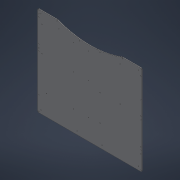
# Autodesk Inventor part: riglt_plate_01
Saved by Autodesk Inventor 2022 (Build 260153000, 153)
## iProperties
Created: 2025-01-09
Part Number: riglt_plate_01
Material: 一般
Document SubType Name: Modeling
Designer: nyxeon
Density: 1 g/cm^3
Appearance: 既定
Author: nyxeon
Autodesk Inventor part; units mm, degrees
ref_plane "YZ Plane" through (0, 0, 0) normal (1, 0, 0) x (0, 1, 0)
ref_plane "XZ Plane" through (0, 0, 0) normal (0, 1, 0) x (-1, 0, 0)
ref_plane "XY Plane" through (0, 0, 0) normal (0, 0, 1) x (1, 0, 0)
sketch "スケッチ1" plane through (0, 0, 0) normal (0, 0, 1) x (1, 0, 0)
  circle A0 centre (233.68, 2.54) radius 2.25 construction
  circle A1 centre (161.29, 2.54) radius 2.25 construction
  circle A2 centre (29.21, 2.54) radius 2.25 construction
  circle A3 centre (233.68, 160.02) radius 2.25 construction
  circle A4 centre (161.29, 160.02) radius 2.25 construction
  circle A5 centre (6.35, 160.02) radius 2.25 construction
  circle A6 centre (6.35, 284.48) radius 2.25 construction
  circle A7 centre (161.29, 284.48) radius 2.25 construction
  circle A8 centre (233.68, 284.48) radius 2.25 construction
  circle A9 centre (29.21, 2.54) radius 1.6
  circle A10 centre (161.29, 2.54) radius 1.6
  circle A11 centre (233.68, 2.54) radius 1.6
  circle A12 centre (233.68, 160.02) radius 1.6
  circle A13 centre (161.29, 160.02) radius 1.6
  circle A14 centre (6.35, 160.02) radius 1.6
  circle A15 centre (6.35, 284.48) radius 1.6
  circle A16 centre (161.29, 284.48) radius 1.6
  circle A17 centre (233.68, 284.48) radius 1.6
  line L0 (495.19, -98.01) -> (-14.81, -98.01)
  line L1 (-14.81, -98.01) -> (-14.81, 311.99)
  line L2 (-14.81, 311.99) -> (495.19, 311.99)
  line L3 (495.19, 311.99) -> (495.19, -98.01)
  line L4 (490.19, 306.99) -> (-9.81, 306.99) construction
  line L5 (-9.81, 306.99) -> (-9.81, -93.01) construction
  line L6 (-9.81, -93.01) -> (490.19, -93.01) construction
  line L7 (490.19, -93.01) -> (490.19, 306.99) construction
  circle A18 centre (-9.81, 306.99) radius 2.1
  circle A19 centre (490.19, 306.99) radius 2.1
  circle A20 centre (490.19, -93.01) radius 2.1
  circle A21 centre (-9.81, -93.01) radius 2.1
  circle A22 centre (-9.81, 6.99) radius 2.1
  circle A23 centre (-9.81, 106.99) radius 2.1
  circle A24 centre (-9.81, 206.99) radius 2.1
  circle A25 centre (90.19, 306.99) radius 2.1
  circle A26 centre (190.19, 306.99) radius 2.1
  circle A27 centre (290.19, 306.99) radius 2.1
  circle A28 centre (390.19, 306.99) radius 2.1
  line L8 (490.19, 106.99) -> (-9.81, 106.99) construction
  line L9 (240.19, -93.01) -> (240.19, 306.99) construction
  circle A29 centre (90.19, -93.01) radius 2.1
  circle A30 centre (190.19, -93.01) radius 2.1
  circle A31 centre (290.19, -93.01) radius 2.1
  circle A32 centre (390.19, -93.01) radius 2.1
  circle A33 centre (490.19, 6.99) radius 2.1
  circle A34 centre (490.19, 106.99) radius 2.1
  circle A35 centre (490.19, 206.99) radius 2.1
  point P0 (0, 0)
  point P1 (-3.81, 297.18)
  point P2 (0, 300.99)
  point P3 (3.7629, -59.9187)
  point P4 (-9.81, 106.99)
  dimension "d0" = 3.2
  dimension "d1" = 510
  dimension "d2" = 410
  dimension "d3" = 11
  dimension "d4" = 11
  dimension "d5" = 5
  dimension "d6" = 4.2
  dimension "d7" = 4.2
  dimension "d8" = 4.2
  dimension "d9" = 4.2
  dimension "d10" = 100
  dimension "d11" = 100
  dimension "d13" = 100
  dimension "d14" = 100
  dimension "d15" = 100
  dimension "d16" = 100
  dimension "d17" = 100
  dimension "d18" = 100
  dimension "d19" = 100
  dimension "d23" = 4.2
  dimension "d24" = 4.2
  dimension "d25" = 4.2
  dimension "d26" = 100
  dimension "d27" = 100
  dimension "d55" = 100
  constraints: 27 centre point, 20 end point, 19 equal radius, 13 coincident, 6 point on line, 5 horizontal alignment, 5 midpoint, 4 parallel, 4 vertical alignment, 2 perpendicular, 1 horizontal, 6 other
  measures "d0" diameter of A9
  measures "d1" distance of L1.end L2.end
  measures "d2" distance of L0.end L1.end
  measures "d3" distance from line of point (-3.81, 297.18) L1
  measures "d4" distance from line of L2 point (0, 300.99)
  measures "d5" distance between parallel lines of L2 L4
  measures "d6" diameter of A21
  measures "d7" diameter of A22
  measures "d8" diameter of A23
  measures "d9" diameter of A24
  measures "d10" distance of A22.centre L5.end
  measures "d11" distance of L8.end A22.centre
  measures "d13" distance of A18.centre A25.centre
  measures "d14" distance of A25.centre A26.centre
  measures "d15" distance of A26.centre A27.centre
  measures "d16" distance of A27.centre A28.centre
  measures "d17" distance of A29.centre A30.centre
  measures "d18" distance of A30.centre A31.centre
  measures "d19" distance of A31.centre A32.centre
  measures "d23" diameter of A33
  measures "d24" diameter of A34
  measures "d25" diameter of A35
  measures "d26" distance of A34.centre A33.centre
  measures "d27" distance of A35.centre A34.centre
  measures "d55" distance of A24.centre L8.end
extrude "押し出し1" add sketch "スケッチ1" along normal blind 3
fillet "フィレット1" radius 5 4 edges at (495.19, -98.01, 1.5) (-14.81, -98.01, 1.5) (-14.81, 311.99, 1.5) (495.19, 311.99, 1.5)
sketch "スケッチ2" plane through (0, 0, 3) normal (0, 0, 1) x (1, 0, 0)
  line L0 (-6.934, 160.0686) -> (-6.134, 160.0686) construction
  line L1 (-6.134, 160.0686) -> (-6.134, 170.6186) construction
  line L2 (-6.134, 170.6186) -> (-6.934, 170.6186) construction
  line L3 (-6.934, 170.6186) -> (-6.934, 160.0686) construction
  line L4 (-6.934, 159.9686) -> (-6.134, 159.9686) construction
  line L5 (-6.134, 170.7186) -> (-6.934, 170.7186)
  arc A0 (-7.334, 161.353) -> (-6.934, 159.9686) centre (-6.934, 160.7186) ccw
  line L6 (-5.734, 159.9686) -> (-5.734, 170.7186) construction
  arc A1 (-6.934, 170.7186) -> (-7.334, 169.3342) centre (-6.934, 169.9686) ccw
  line L7 (-7.334, 161.353) -> (-7.334, 169.3342)
  arc A2 (-6.134, 159.9686) -> (-6.134, 161.4686) centre (-6.134, 160.7186) ccw construction
  arc A3 (-6.134, 169.2186) -> (-6.134, 170.7186) centre (-6.134, 169.9686) ccw construction
  arc A4 (-6.134, 159.9686) -> (-5.734, 161.353) centre (-6.134, 160.7186) ccw
  arc A5 (-5.734, 169.3342) -> (-6.134, 170.7186) centre (-6.134, 169.9686) ccw
  line L8 (-5.734, 161.353) -> (-5.734, 169.3342)
  line L9 (-6.934, 159.9686) -> (-6.134, 159.9686)
  line L10 (-7.334, 181.753) -> (-7.334, 189.7342)
  arc A6 (-7.334, 181.753) -> (-6.934, 180.3686) centre (-6.934, 181.1186) ccw
  arc A7 (-6.134, 180.3686) -> (-5.734, 181.753) centre (-6.134, 181.1186) ccw
  line L11 (-5.734, 181.753) -> (-5.734, 189.7342)
  line L12 (-6.934, 180.3686) -> (-6.134, 180.3686)
  arc A8 (-6.934, 191.1186) -> (-7.334, 189.7342) centre (-6.934, 190.3686) ccw
  line L13 (-6.134, 191.1186) -> (-6.934, 191.1186)
  arc A9 (-5.734, 189.7342) -> (-6.134, 191.1186) centre (-6.134, 190.3686) ccw
  line L14 (-7.334, 202.153) -> (-7.334, 210.1342)
  arc A10 (-7.334, 202.153) -> (-6.934, 200.7686) centre (-6.934, 201.5186) ccw
  arc A11 (-6.134, 200.7686) -> (-5.734, 202.153) centre (-6.134, 201.5186) ccw
  line L15 (-5.734, 202.153) -> (-5.734, 210.1342)
  line L16 (-6.934, 200.7686) -> (-6.134, 200.7686)
  arc A12 (-6.934, 211.5186) -> (-7.334, 210.1342) centre (-6.934, 210.7686) ccw
  line L17 (-6.134, 211.5186) -> (-6.934, 211.5186)
  arc A13 (-5.734, 210.1342) -> (-6.134, 211.5186) centre (-6.134, 210.7686) ccw
  line L18 (-7.334, 222.553) -> (-7.334, 230.5342)
  arc A14 (-7.334, 222.553) -> (-6.934, 221.1686) centre (-6.934, 221.9186) ccw
  arc A15 (-6.134, 221.1686) -> (-5.734, 222.553) centre (-6.134, 221.9186) ccw
  line L19 (-5.734, 222.553) -> (-5.734, 230.5342)
  line L20 (-6.934, 221.1686) -> (-6.134, 221.1686)
  arc A16 (-6.934, 231.9186) -> (-7.334, 230.5342) centre (-6.934, 231.1686) ccw
  line L21 (-6.134, 231.9186) -> (-6.934, 231.9186)
  arc A17 (-5.734, 230.5342) -> (-6.134, 231.9186) centre (-6.134, 231.1686) ccw
  line L22 (-7.334, 242.953) -> (-7.334, 250.9342)
  arc A18 (-7.334, 242.953) -> (-6.934, 241.5686) centre (-6.934, 242.3186) ccw
  arc A19 (-6.134, 241.5686) -> (-5.734, 242.953) centre (-6.134, 242.3186) ccw
  line L23 (-5.734, 242.953) -> (-5.734, 250.9342)
  line L24 (-6.934, 241.5686) -> (-6.134, 241.5686)
  arc A20 (-6.934, 252.3186) -> (-7.334, 250.9342) centre (-6.934, 251.5686) ccw
  line L25 (-6.134, 252.3186) -> (-6.934, 252.3186)
  arc A21 (-5.734, 250.9342) -> (-6.134, 252.3186) centre (-6.134, 251.5686) ccw
  line L26 (-7.334, 263.353) -> (-7.334, 271.3342)
  arc A22 (-7.334, 263.353) -> (-6.934, 261.9686) centre (-6.934, 262.7186) ccw
  arc A23 (-6.134, 261.9686) -> (-5.734, 263.353) centre (-6.134, 262.7186) ccw
  line L27 (-5.734, 263.353) -> (-5.734, 271.3342)
  line L28 (-6.934, 261.9686) -> (-6.134, 261.9686)
  arc A24 (-6.934, 272.7186) -> (-7.334, 271.3342) centre (-6.934, 271.9686) ccw
  line L29 (-6.134, 272.7186) -> (-6.934, 272.7186)
  arc A25 (-5.734, 271.3342) -> (-6.134, 272.7186) centre (-6.134, 271.9686) ccw
  line L30 (-7.334, 283.753) -> (-7.334, 291.7342)
  arc A26 (-7.334, 283.753) -> (-6.934, 282.3686) centre (-6.934, 283.1186) ccw
  arc A27 (-6.134, 282.3686) -> (-5.734, 283.753) centre (-6.134, 283.1186) ccw
  line L31 (-5.734, 283.753) -> (-5.734, 291.7342)
  line L32 (-6.934, 282.3686) -> (-6.134, 282.3686)
  arc A28 (-6.934, 293.1186) -> (-7.334, 291.7342) centre (-6.934, 292.3686) ccw
  line L33 (-6.134, 293.1186) -> (-6.934, 293.1186)
  arc A29 (-5.734, 291.7342) -> (-6.134, 293.1186) centre (-6.134, 292.3686) ccw
  point P0 (0, 0)
  point P1 (-6.934, 180.4686)
  point P2 (-6.134, 191.0186)
  dimension "d34" = 20.4
  dimension "d37" = 1.5
  dimension "d39" = 0.1
  dimension "d40" = 0.1
  dimension "d41" = 1.6
  dimension "d42" = 0.8
  dimension "d43" = 0.4
  dimension "d46" = 20.4
  constraints: 68 end point, 62 point on circle, 30 centre point, 4 parallel, 4 tangent, 4 vertical alignment, 3 equal radius, 2 coincident, 2 horizontal alignment, 2 point on line, 2 vertical, 1 collinear, 1 horizontal, 1 perpendicular, 124 other
  measures "d34" distance of point (-6.934, 180.469) L0.start
  measures "d37" diameter of A0
  measures "d39" distance between parallel lines of L0 L4
  measures "d40" distance between parallel lines of L2 L5
  measures "d41" distance between parallel lines of L8 L7
  measures "d42" horizontal distance of L1.end L0.start
  measures "d43" distance between parallel lines of L3 L7
  measures "d46" distance of L7.start L10.start
extrude "押し出し2" [suppressed]
sketch "スケッチ6" plane through (0, 0, 3) normal (0, 0, 1) x (1, 0, 0)
  arc A0 (379.99, -128.01) -> (100.39, -128.01) centre (240.19, -438.744) ccw
  arc A1 (483.7257, -128.01) -> (483.7257, 341.99) centre (-161.4767, 106.99) ccw
  arc A2 (79.99, 341.99) -> (400.39, 341.99) centre (240.19, 754.724) ccw
  arc A3 (-3.3457, 341.99) -> (-3.3457, -128.01) centre (641.8567, 106.99) ccw
  line L0 (-9.81, -98.01) -> (490.19, -98.01) projected
  arc A4 (490.19, -98.01) -> (495.19, -93.01) centre (490.19, -93.01) ccw projected
  line L1 (495.19, -93.01) -> (495.19, 306.99) projected
  arc A5 (495.19, 306.99) -> (490.19, 311.99) centre (490.19, 306.99) ccw projected
  line L2 (490.19, 311.99) -> (-9.81, 311.99) projected
  arc A6 (-9.81, 311.99) -> (-14.81, 306.99) centre (-9.81, 306.99) ccw projected
  line L3 (-14.81, 306.99) -> (-14.81, -93.01) projected
  arc A7 (-14.81, -93.01) -> (-9.81, -98.01) centre (-9.81, -93.01) ccw projected
  line L4 (483.7257, -128.01) -> (379.99, -128.01)
  line L5 (100.39, -128.01) -> (-3.3457, -128.01)
  line L6 (483.7257, 341.99) -> (400.39, 341.99)
  line L7 (79.99, 341.99) -> (-3.3457, 341.99)
  point P0 (0, 0)
  point P1 (-14.59, 308.457)
  point P2 (-14.59, -94.477)
  point P3 (494.97, -94.477)
  point P4 (494.97, 308.457)
  point P5 (240.19, 311.99)
  point P6 (240.19, -98.01)
  constraints: 8 end point, 8 point on circle, 4 centre point, 2 collinear, 1 horizontal, 1 parallel, 16 other
extrude "押し出し5" add sketch "スケッチ6" against normal up to surface (3 mm away) contours A5 L2 A2 L6 A1 | A3 L7 A2 L2 A6
sketch "スケッチ7" plane through (0, 0, 3) normal (0, 0, 1) x (1, 0, 0)
  arc A0 (495.19, 306.99) -> (494.97, 308.457) centre (490.19, 306.99) ccw projected
  arc A1 (494.97, 308.457) -> (483.7257, 341.99) centre (-161.4767, 106.99) ccw projected
  arc A2 (-3.3457, 341.99) -> (-14.59, 308.457) centre (641.8567, 106.99) ccw projected
  arc A3 (-14.59, 308.457) -> (-14.81, 306.99) centre (-9.81, 306.99) ccw projected
  line L0 (-14.81, 306.99) -> (-14.81, 336.99)
  line L1 (-9.81, 341.99) -> (-3.3457, 341.99)
  arc A4 (495.19, 306.99) -> (494.97, 308.457) centre (490.19, 306.99) ccw projected
  line L2 (495.19, 306.99) -> (495.19, 336.99)
  line L3 (483.7257, 341.99) -> (400.39, 341.99) projected
  line L4 (490.19, 341.99) -> (483.7257, 341.99)
  arc A5 (-9.81, 341.99) -> (-14.81, 336.99) centre (-9.81, 336.99) ccw
  arc A6 (495.19, 336.99) -> (490.19, 341.99) centre (490.19, 336.99) ccw
  point P0 (0, 0)
  point P1 (-14.81, 341.99)
  point P2 (495.19, 341.99)
  dimension "d62" = 5
  constraints: 8 end point, 5 tangent, 4 point on circle, 4 point on line, 2 centre point, 2 perpendicular, 2 vertical, 1 equal radius
  measures "d62" radius of A5
extrude "押し出し6" add sketch "スケッチ7" against normal up to surface (3 mm away)
fillet "フィレット2" radius 5 2 edges at (400.39, 341.99, 1.5) (79.99, 341.99, 1.5)
sketch "スケッチ8" plane through (0, 0, 3) normal (0, 0, 1) x (1, 0, 0)
  circle A0 centre (490.19, -93.01) radius 2.1 construction
  circle A1 centre (-9.81, -93.01) radius 2.1 construction
  arc A2 (-9.81, 341.99) -> (-14.81, 336.99) centre (-9.81, 336.99) ccw construction
  arc A3 (495.19, 336.99) -> (490.19, 341.99) centre (490.19, 336.99) ccw construction
  circle A4 centre (479.19, -82.01) radius 2.1
  circle A5 centre (1.19, -82.01) radius 2.1
  circle A6 centre (1.19, 325.99) radius 2.1
  circle A7 centre (479.19, 325.99) radius 2.1
  circle A8 centre (490.19, 336.99) radius 2.1
  circle A9 centre (-9.81, 336.99) radius 2.1
  arc A10 (401.3236, 341.99) -> (399.5242, 341.655) centre (401.3236, 336.99) ccw construction
  arc A11 (80.8558, 341.655) -> (79.0564, 341.99) centre (79.0564, 336.99) ccw construction
  circle A12 centre (79.0564, 336.99) radius 2.1
  circle A13 centre (401.3236, 336.99) radius 2.1
  point P0 (0, 0)
  dimension "d63" = 11
  dimension "d64" = 11
  dimension "d65" = 11
  dimension "d66" = 11
  dimension "d67" = 11
  dimension "d68" = 11
  dimension "d69" = 11
  dimension "d70" = 11
  constraints: 8 centre point, 8 equal radius, 4 coincident
  measures "d63" horizontal distance of A4.centre A0.centre
  measures "d64" horizontal distance of A4.centre A0.centre
  measures "d65" horizontal distance of A1.centre A5.centre
  measures "d66" horizontal distance of A1.centre A5.centre
  measures "d67" horizontal distance of A2.centre A6.centre
  measures "d68" horizontal distance of A2.centre A6.centre
  measures "d69" horizontal distance of A7.centre A3.centre
  measures "d70" horizontal distance of A3.centre A7.centre
extrude "押し出し7" cut sketch "スケッチ8" against normal through all
sketch "スケッチ9" plane through (0, 0, 0) normal (0, 0, -1) x (-1, 0, 0)
  circle A0 centre (-490.19, 6.99) radius 2.1 construction
  line L0 (-490.19, 6.99) -> (-490.19, -23.01) construction
  circle A1 centre (-490.19, -23.01) radius 2.1
  circle A2 centre (-490.19, 106.99) radius 2.1 construction
  line L1 (-490.19, 106.99) -> (-490.19, 136.99) construction
  circle A3 centre (-490.19, 136.99) radius 2.1
  circle A4 centre (9.81, 206.99) radius 2.1 construction
  line L2 (9.81, 206.99) -> (9.81, 176.99) construction
  circle A5 centre (9.81, 176.99) radius 2.1
  circle A6 centre (-490.19, 121.99) radius 2.1
  circle A7 centre (9.81, 191.99) radius 2.1
  circle A8 centre (9.81, 161.99) radius 2.1
  circle A9 centre (9.81, 306.99) radius 2.1 construction
  circle A10 centre (9.81, 336.99) radius 2.1 construction
  circle A11 centre (9.81, 336.99) radius 2.1 construction
  line L3 (9.81, 306.99) -> (9.81, 336.99) construction
  circle A12 centre (9.81, 321.99) radius 2.1
  circle A13 centre (-490.19, -8.01) radius 2.1
  circle A14 centre (9.81, 6.99) radius 2.1 construction
  line L4 (9.81, 6.99) -> (9.81, -23.01) construction
  circle A15 centre (9.81, -23.01) radius 2.1
  point P0 (0, 0)
  dimension "d74" = 30
  dimension "d77" = 15
  dimension "d78" = 30
  constraints: 10 end point, 9 centre point, 9 equal radius, 5 vertical, 4 coincident, 4 midpoint, 2 equal length, 1 vertical alignment
  measures "d74" distance of L0.start L0.end
  measures "d77" distance of L2.end A8.centre
  measures "d78" distance of L4.start L4.end
extrude "押し出し8" cut sketch "スケッチ9" against normal through all
sketch "スケッチ10" plane through (0, 0, 3) normal (0, 0, 1) x (1, 0, 0)
  circle A0 centre (290.19, -93.01) radius 2.1 construction
  circle A1 centre (190.19, -93.01) radius 2.1 construction
  circle A2 centre (479.19, -82.01) radius 2.1 construction
  circle A3 centre (1.19, -82.01) radius 2.1 construction
  circle A4 centre (301.19, -82.01) radius 2.1
  circle A5 centre (179.19, -82.01) radius 2.1
  line L0 (479.19, -82.01) -> (1.19, -82.01) construction
  point P0 (0, 0)
  dimension "d79" = 11
  dimension "d80" = 11
  dimension "d81" = 11
  dimension "d82" = 11
  constraints: 2 centre point, 2 end point, 2 equal radius, 1 horizontal
  measures "d79" horizontal distance of A0.centre A4.centre
  measures "d80" horizontal distance of A4.centre A0.centre
  measures "d81" horizontal distance of A5.centre A1.centre
  measures "d82" horizontal distance of A5.centre A1.centre
extrude "押し出し9" cut sketch "スケッチ10" against normal up to surface (3 mm away)
sketch "スケッチ11" plane through (0, 0, 3) normal (0, 0, 1) x (1, 0, 0)
  circle A0 centre (490.19, 106.99) radius 2.1 projected
  circle A1 centre (-9.81, 206.99) radius 2.1 projected
  circle A2 centre (-9.81, 106.99) radius 2.1 projected
  circle A3 centre (-9.81, 6.99) radius 2.1 projected
  circle A4 centre (90.19, -93.01) radius 2.1 projected
  circle A5 centre (190.19, -93.01) radius 2.1 projected
  circle A6 centre (290.19, -93.01) radius 2.1 projected
  circle A7 centre (390.19, -93.01) radius 2.1 projected
  circle A8 centre (90.19, 306.99) radius 2.1 projected
  point P0 (0, 0)
extrude "押し出し10" add sketch "スケッチ11" against normal up to surface (3 mm away)
sketch "スケッチ12" plane through (0, 0, 3) normal (0, 0, 1) x (1, 0, 0)
  circle A0 centre (490.19, 6.99) radius 2.1 construction
  circle A1 centre (490.19, 136.99) radius 2.1 construction
  circle A2 centre (490.19, 206.99) radius 2.1 construction
  circle A3 centre (290.19, 306.99) radius 2.1 construction
  circle A4 centre (390.19, 306.99) radius 2.1 construction
  circle A5 centre (390.19, 6.99) radius 2.1
  circle A6 centre (290.19, 6.99) radius 2.1
  circle A7 centre (390.19, 136.99) radius 2.1
  circle A8 centre (290.19, 136.99) radius 2.1
  point P0 (0, 0)
  constraints: 4 centre point, 4 equal radius, 4 horizontal alignment, 4 vertical alignment
extrude "押し出し11" cut sketch "スケッチ12" against normal up to surface (3 mm away) contours A6 | A7 | A8
equation "\"d10\" = -0.5 * d5 + 0.25 * d2"
equation "\"d11\" = d10"
equation "\"d13\" = -0.4 * d5 + 0.2 * d1"
equation "\"d14\" = d13"
equation "\"d15\" = d13"
equation "\"d16\" = d13"
equation "\"d17\" = d20"
equation "\"d18\" = d20"
equation "\"d19\" = d20"
equation "\"d26\" = d28"
equation "\"d27\" = d26"
equation "\"d40\" = d39"
equation "\"d43\" = -0.5 * d42 + 0.5 * d41"
equation "\"d46\" = d34"
equation "\"d65\" = d63"
equation "\"d66\" = d63"
equation "\"d67\" = d63"
equation "\"d68\" = d63"
equation "\"d69\" = d63"
equation "\"d70\" = d63"
equation "\"d77\" = 0.5 * d74"
equation "\"d79\" = d4"
equation "\"d80\" = d79"
equation "\"d81\" = d79"
equation "\"d82\" = d80"
equation "\"d20\" = -0.4 * d22 + 0.2 * d21"
equation "\"d28\" = -0.5 * d30 + 0.25 * d29"
equation "\"d22\" = 5"
equation "\"d21\" = 510"
equation "\"d30\" = 5"
equation "\"d29\" = 410"
